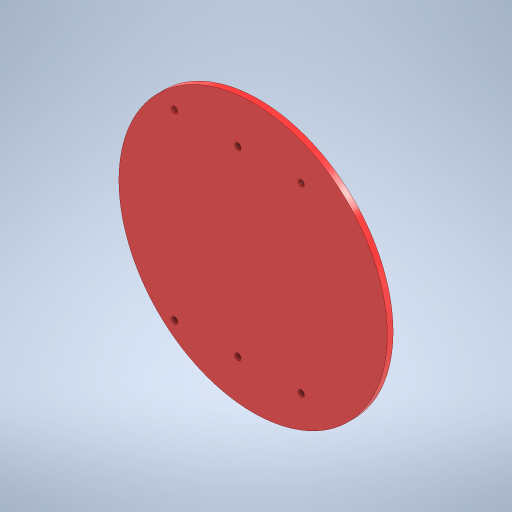
# Autodesk Inventor part: фанера для акб
Saved by Autodesk Inventor 2023 (Build 270158000, 158)
## iProperties
Created: 2024-03-01
Part Number: фанера для акб
Material: Типовые
Document SubType Name: Modeling
Designer: liza
Density: 1 g/cm^3
Appearance: Светло-красный
Author: liza
Autodesk Inventor part; units mm, degrees
ref_plane "YZ Plane" through (0, 0, 0) normal (1, 0, 0) x (0, 1, 0)
ref_plane "XZ Plane" through (0, 0, 0) normal (0, 1, 0) x (-1, 0, 0)
ref_plane "XY Plane" through (0, 0, 0) normal (0, 0, 1) x (1, 0, 0)
sketch "Эскиз1" plane through (0, 0, 0) normal (0, 0, 1) x (1, 0, 0)
  circle A0 centre (0, 0) radius 70
  circle A1 centre (-40.8825, 46.3163) radius 1.6 projected
  circle A2 centre (-7.8825, 46.3163) radius 1.6 projected
  circle A3 centre (25.1173, 46.3164) radius 1.6002 projected
  circle A4 centre (25.1175, -48.6837) radius 1.6 projected
  circle A5 centre (-7.8825, -48.6837) radius 1.6 projected
  circle A6 centre (-40.8826, -48.6837) radius 1.6001 projected
  dimension "d0" = 140
  constraints: 1 centre point, 1 coincident
  measures "d0" diameter of A0
extrude "Выдавливание1" add sketch "Эскиз1" along normal blind 3 contours A0 | A1 | A2 | A3 | A4 | A5 | A6
sketch "Эскиз3" plane through (0, 0, 0) normal (0, 0, -1) x (-1, 0, 0)
  circle A0 centre (40.8825, -48.6837) radius 1.6 projected
  circle A1 centre (7.8825, -48.6837) radius 1.6001 projected
  circle A2 centre (-25.1176, -48.684) radius 1.5997 projected
  circle A3 centre (-25.1178, 46.3162) radius 1.5997 projected
  circle A4 centre (7.8825, 46.3163) radius 1.6001 projected
  circle A5 centre (40.8824, 46.3162) radius 1.5999 projected
  point P0 (0, 0)
extrude "Выдавливание2" cut sketch "Эскиз3" against normal through all
